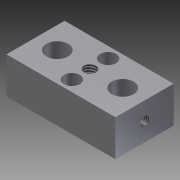
# Autodesk Inventor part: 13_0204_020
Saved by Autodesk Inventor 2012 SP1 (Build 160190100, 190)
## iProperties
Created: 2013-03-27
Part Number: 13_0204_020
Material: Default
Document SubType Name: Modeling
Designer: vogel
Density: 1 g/cm^3
Author: vogel
Autodesk Inventor part; units mm, degrees
note: some values were not read from the file. Chosen so that the rebuilt part matches the saved one: direction of "Bohrung4".
ref_plane "YZ Plane" through (0, 0, 0) normal (1, 0, 0) x (0, 1, 0)
ref_plane "XZ Plane" through (0, 0, 0) normal (0, 1, 0) x (-1, 0, 0)
ref_plane "XY Plane" through (0, 0, 0) normal (0, 0, 1) x (1, 0, 0)
sketch "Skizze1" plane through (0, 0, 0) normal (0, 0, 1) x (1, 0, 0)
  line L0 (-15, 8) -> (15, 8)
  line L1 (15, 8) -> (15, -8)
  line L2 (15, -8) -> (-15, -8)
  line L3 (-15, -8) -> (-15, 8)
  line L4 (-21, 0) -> (21, 0) projected
  line L5 (0, -11.2) -> (0, 11.2) projected
  point P0 (0, 0)
  dimension "d0" = 16
  dimension "d1" = 30
  constraints: 8 end point, 2 parallel, 1 horizontal, 1 perpendicular, 2 other
  measures "d0" distance of L2.end L0.start
  measures "d1" distance of L1.end L2.end
extrude "Extrusion1" add sketch "Skizze1" along normal blind 10
sketch "Skizze2" plane through (0, 0, 10) normal (0, 0, 1) x (1, 0, 0)
  line L0 (-21, 0) -> (21, 0) projected
  line L1 (0, -11.2) -> (0, 11.2) projected
  point P0 (0, 0)
  point P1 (-9, 0)
  point P2 (9, 0)
  dimension "d4" = 18
  constraints: 2 point on line, 1 symmetric about line
  measures "d4" distance of point (9, 0) point (-9, 0)
hole "Bohrung1" at (-9, 0, 10) at (9, 0, 10) direction (0, 0, -1) diameter 6 end through all
sketch "Skizze3" plane through (0, 0, 10) normal (0, 0, 1) x (1, 0, 0)
  line L0 (0, -11.2) -> (0, 11.2) projected
  line L1 (-21, 0) -> (21, 0) projected
  point P0 (0, 0)
  point P1 (0, 5)
  point P2 (0, -5)
  dimension "d12" = 10
  constraints: 2 point on line, 1 symmetric about line
  measures "d12" distance of point (0, -5) point (0, 5)
hole "Bohrung2" at (0, 5, 10) at (0, -5, 10) direction (0, 0, -1) diameter 2.3 end through all counterbore diameter 4.4 counterbore depth 6
sketch "Skizze4" plane through (0, 0, 10) normal (0, 0, 1) x (1, 0, 0)
  point P0 (0, 0)
  point P1 (0, 0)
  constraints: 1 coincident
hole "Bohrung3" at (0, 0, 10) direction (0, 0, -1) diameter 3.242 end through all thread size "M4x0.7" class "6H" standard "ISO Metric profile"
sketch "Skizze5" plane through (-15, -8, 0) normal (-1, 0, 0) x (0, 0, 1)
  line L0 (10, 0) -> (10, 16) projected
  line L1 (0, 16) -> (10, 16) projected
  line L2 (0, 0) -> (10, 0) projected
  line L3 (0, 8) -> (10, 8)
  line L4 (5, 16) -> (5, 0)
  point P0 (5, 8)
  constraints: 4 end point, 4 midpoint
hole "Bohrung4" at (-15, 0, 5) direction (1, 0, 0) diameter 2.459 end up to surface thread size "M3x0.5" class "6H" standard "ISO Metric profile"
mirror "Spiegeln1" about plane through (0, 0, 0) normal (1, 0, 0) of "Bohrung4"
